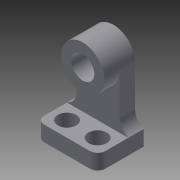
# Autodesk Inventor part: 7.1 Part 5
Saved by Autodesk Inventor 2015 (Build 190159000, 159)
## iProperties
Created: 2015-03-05
Part Number: 7.1 Part 5
Material: Generic
Document SubType Name: Modeling
Designer: PLTW-Stu-02
Density: 1 g/cm^3
Appearance: Default
Author: PLTW-Stu-02
Autodesk Inventor part; units mm, degrees
ref_plane "YZ Plane" through (0, 0, 0) normal (1, 0, 0) x (0, 1, 0)
ref_plane "XZ Plane" through (0, 0, 0) normal (0, 1, 0) x (-1, 0, 0)
ref_plane "XY Plane" through (0, 0, 0) normal (0, 0, 1) x (1, 0, 0)
sketch "Sketch1" plane through (0, 0, 0) normal (0, 1, 0) x (-1, 0, 0)
  line L0 (6.9046, -9.2909) -> (57.7046, -9.2909)
  line L1 (57.7046, -9.2909) -> (57.7046, -47.3909)
  line L2 (57.7046, -47.3909) -> (6.9046, -47.3909)
  line L3 (6.9046, -47.3909) -> (6.9046, -9.2909)
  point P0 (0, 0)
  dimension "d0" = 50.8
  dimension "d1" = 38.1
  constraints: 8 end point, 2 parallel, 1 horizontal, 1 perpendicular
  measures "d0" distance of L1.end L2.end
  measures "d1" distance of L0.end L1.end
extrude "Extrusion1" add sketch "Sketch1" along normal blind 12.7
fillet "Fillet1" radius 6.35 2 edges at (-6.9046, 6.35, -9.2909) (-57.7046, 6.35, -9.2909)
sketch "Sketch2" plane through (0, 12.7, 0) normal (0, 1, 0) x (1, 0, 0)
  point P0 (0, 0)
  point P1 (-19.6046, 21.9909)
  point P2 (-45.0046, 21.9909)
sketch "Sketch3" plane through (0, 12.7, 0) normal (0, 1, 0) x (1, 0, 0)
  line L0 (-6.9046, 47.3909) -> (-6.9046, 15.6409) projected
  line L1 (-57.7046, 47.3909) -> (-6.9046, 47.3909)
  line L2 (-6.9046, 47.3909) -> (-6.9046, 34.6909)
  line L3 (-6.9046, 34.6909) -> (-57.7046, 34.6909)
  line L4 (-57.7046, 34.6909) -> (-57.7046, 47.3909)
  point P0 (0, 0)
  dimension "d16" = 12.7
  constraints: 8 end point, 2 parallel, 1 horizontal, 1 perpendicular, 1 point on line
  measures "d16" distance of L1.end L2.end
extrude "Extrusion2" add sketch "Sketch3" along normal blind 63.5
sketch "Sketch4" plane through (-57.7046, 12.7, -34.6909) normal (0, 0, 1) x (1, 0, 0)
  line L0 (0, 0) -> (6.35, 0) projected
  arc A0 (43.7412, 12.7) -> (50.8, 0) centre (56.3756, 11.4106) ccw
  line L1 (43.7412, 12.7) -> (43.7412, 44.45)
  line L2 (44.45, 0) -> (50.8, 0) projected
  arc A1 (0, 0) -> (7.8514, 12.7) centre (-4.8133, 11.7526) ccw
  line L3 (7.8514, 12.7) -> (7.8514, 44.45)
  circle A2 centre (25.7961, 44.45) radius 17.9451
  circle A3 centre (25.7961, 44.45) radius 9.525
  line L4 (0, 0) -> (50.8, 0)
  arc A4 (43.7412, 44.45) -> (7.8514, 44.45) centre (25.7963, 44.45) ccw
  arc A5 (7.8514, 44.45) -> (43.7412, 44.45) centre (25.7963, 44.45) ccw
  line L5 (0, 0) -> (0, 63.5)
  line L6 (0, -12.7) -> (0, 63.5) projected
  line L7 (0, 63.5) -> (50.8, 63.5)
  line L8 (50.8, 63.5) -> (50.8, 0)
  line L9 (50.8, -12.7) -> (50.8, 63.5) projected
  point P0 (57.7046, -12.7)
  constraints: 12 end point, 8 point on circle, 6 centre point, 4 tangent, 2 collinear, 2 vertical, 1 coincident, 1 perpendicular
extrude "Extrusion3" cut sketch "Sketch4" against normal blind 25.4 contours L5 L7 L8 A0 L1 A2 L3 A1
extrude "Extrusion4" cut sketch "Sketch4" against normal blind 25.4 contours A3
extrude "Extrusion5" add sketch "Sketch4" along normal blind 12.7 contours A2
hole "Hole2" at (-19.6046, 12.7, -21.9909) at (-45.0046, 12.7, -21.9909) direction (0, -1, 0) diameter 15.24 end through all
body "Solid1"
